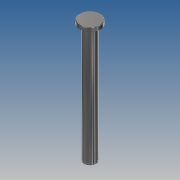
# Autodesk Inventor part: DD_KVD_003_10_B
Saved by Autodesk Inventor 2017.3 (Build 213256000, 256)
## iProperties
Created: 2023-12-12
Part Number: DD_KVD_003_10_B
Material: Nerezová ocel
Document SubType Name: Modeling
Designer: Darena
Manufacturer: Standard
Standards Organization: Custom
Density: 8 g/cm^3
Appearance: Pololeštěná
Author: Darena
Autodesk Inventor part; units mm, degrees
ref_plane "YZ Plane" through (0, 0, 0) normal (1, 0, 0) x (0, 1, 0)
ref_plane "XZ Plane" through (0, 0, 0) normal (0, 1, 0) x (-1, 0, 0)
ref_plane "XY Plane" through (0, 0, 0) normal (0, 0, 1) x (1, 0, 0)
sketch "Náčrt2" plane through (0, 0, 0) normal (1, 0, 0) x (0, 1, 0)
  line L0 (0, 0) -> (0, -130.5)
  line L1 (0, 0) -> (11, 0)
  line L2 (11, 0) -> (11, -4)
  line L3 (11, -4) -> (6.5, -4)
  line L4 (6.5, -4) -> (6.5, -127.9)
  line L5 (6.5, -127.9) -> (6.2, -127.9)
  line L6 (6.2, -127.9) -> (6.2, -129)
  line L7 (6.2, -129) -> (6.5, -129)
  line L8 (6.5, -129) -> (6.5, -130.5)
  line L9 (6.5, -130.5) -> (0, -130.5)
  dimension "d0" = 13
  dimension "d1" = 22
  dimension "d3" = 4
  dimension "d4" = 12.4
  dimension "d5" = 1.1
  dimension "d6" = 1.5
  dimension "d11" = 123.9
  dimension "d12" = 130.5
  constraints: 20 end point, 7 perpendicular, 2 point on line, 1 horizontal, 1 vertical
  measures "d0" diameter of L4 L0
  measures "d1" diameter of L2 L0
  measures "d3" distance between parallel lines of L3 L1
  measures "d4" diameter of L6 L0
  measures "d5" distance of L5.end L6.end
  measures "d6" distance of L7.end L8.end
  measures "d11" distance of L3.end L4.end
  measures "d12" distance between parallel lines of L9 L1
revolve "Rotace1" add sketch "Náčrt2" angle 360 about axis through (0, 0, 0) along (0, 0, -1)
chamfer "Zkosení1" distance 0.5 angle 45 2 edges at (0, -11, 0) (0, -6.5, -130.5)
